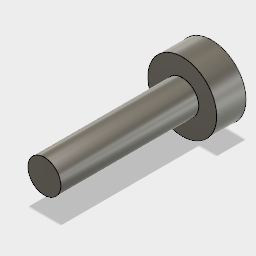
Spool_Holder_and_Filament_Guide (Autodesk Fusion 360 archive; units mm, degrees)
design "3mm with Washer - Loose Fit"
Autodesk Fusion 360 part; units mm, degrees
cylinder "CylinderPrimitive1" add diameter 7.5 height 3.2 placed x (1, 0, 0) y (0, 1, 0) z (0, 0, 1) at (0, 0, 0)
cylinder "CylinderPrimitive2" add diameter 3.6 height 15 placed x (1, 0, 0) y (0, 1, 0) z (0, 0, 1) at (0, 0, 3.2)

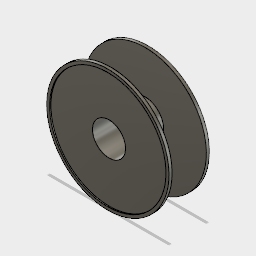
design "Spool"
Autodesk Fusion 360 part; units mm, degrees
sketch "Spool" plane through (0, 0, 0) normal (1, 0, 0) x (0, 0, -1)
  line L0 (33, -100) -> (28, -100)
  line L1 (28, -100) -> (28, -30)
  line L2 (10, 0) -> (0, 0) construction
  line L3 (33, -100) -> (33, -95)
  line L4 (33, -95) -> (31, -95)
  line L5 (31, -95) -> (31, -27)
  line L6 (0, -27) -> (0, -87.6876) construction
  line L7 (0, -27) -> (31, -27)
  line L8 (28, -30) -> (0, -30)
  line L9 (-33, -100) -> (-28, -100)
  line L10 (-28, -100) -> (-28, -30)
  line L11 (-28, -30) -> (0, -30)
  line L12 (0, -27) -> (-31, -27)
  line L13 (-31, -95) -> (-31, -27)
  line L14 (-33, -100) -> (-33, -95)
  line L15 (-33, -95) -> (-31, -95)
  line L16 (0, 10) -> (0, 0) construction
  dimension "d17" = 5
  dimension "d18" = 100
  dimension "d20" = 27
  dimension "d24" = 28
  dimension "d37" = 3
  dimension "d44" = 33
  dimension "d46" = 2
  measures "d17" distance of L0.start L3.end
  measures "d18" distance of L0 L2
  measures "d20" distance of L2 L7
  measures "d24" distance of L1 L6
  measures "d37" distance of L7 L8
  measures "d44" distance of L3 L6
  measures "d46" distance of L3 L5
revolve "Revolve1" add sketch "Spool" angle 360 about axis through (0, 0, -10) along (0, 0, 1)
ref_plane "WorkPlane1" through (0, 0, 0) normal (0, 0, 1) x (1, 0, 0)
equation "d18 = 0.5 * SpoolDia"
equation "d20 = 0.5 * HubDia"
equation "d24 = 0.5 * InsideHeight"
equation "d37 = Thickness"
equation "SpoolDia = 200 mm"
equation "HubDia = 54 mm"
equation "TotalHeight = 66 mm"
equation "d44 = 0.5 * TotalHeight"
equation "LipSize = 2 mm"
equation "d46 = LipSize"
equation "InsideHeight = 56 mm"
equation "Thickness = 0.5 * ( TotalHeight - InsideHeight ) - LipSize"
named bodies: "Spool"

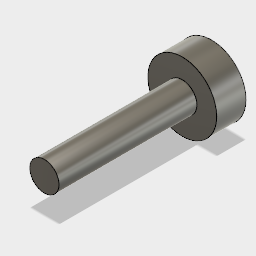
design "3mm with Washer - Close Fit"
Autodesk Fusion 360 part; units mm, degrees
cylinder "CylinderPrimitive1" add diameter 7.5 height 3.2 placed x (1, 0, 0) y (0, 1, 0) z (0, 0, 1) at (0, 0, 0)
cylinder "CylinderPrimitive2" add diameter 3.2 height 15 placed x (1, 0, 0) y (0, 1, 0) z (0, 0, 1) at (0, 0, 3.2)

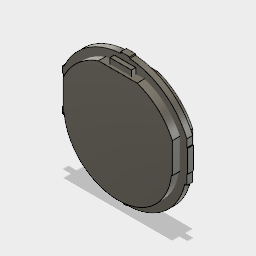
design "RFID Reader Cut Out"
Autodesk Fusion 360 part; units mm, degrees
ref_plane "WorkPlane1" through (3.9732, 4.9722, 0) normal (0, 0, 1) x (1, 0, 0)
sketch "Body Cut for Electronics" plane through (0, 0, 0) normal (0, 0, 1) x (1, 0, 0)
  line L0 (2.1432, 29.163) -> (5.5032, 29.163)
  line L1 (3.8232, 29.163) -> (3.8232, 19.163) construction
  line L2 (7.8232, 29.163) -> (7.8232, 19.163)
  line L3 (-0.1768, 19.163) -> (7.8232, 19.163)
  line L4 (2.1432, 29.163) -> (2.1432, 28.6377)
  line L5 (5.5032, 29.163) -> (5.5032, 28.6548)
  arc A0 (26.7732, 13.4919) -> (5.5032, 28.6548) centre (3.8232, 3.7982) ccw
  arc A1 (2.1432, 28.6377) -> (-18.9127, 13.9615) centre (3.8256, 3.7813) ccw
  line L6 (-0.1768, 26.913) -> (7.8232, 26.913)
  line L7 (-0.1768, 29.163) -> (-0.1768, 19.163)
  dimension "d10" = 10
  dimension "d11" = 4
  measures "d10" distance of L1.start L1.end
sketch "sketch 149" plane through (0, 0, 0) normal (0, 0, 1) x (1, 0, 0)
  line L0 (2.1432, 29.163) -> (2.1432, 28.6377)
  line L1 (5.5032, 29.163) -> (5.5032, 28.6548)
  line L2 (26.7732, 13.4919) -> (26.7732, 10.6115)
  line L3 (26.7732, 2.2615) -> (26.7732, -1.4856)
  line L4 (27.0732, 10.6115) -> (27.0732, 2.2615)
  line L5 (3.0732, -19.1885) -> (3.0732, -18.9361)
  line L6 (4.5732, -19.1885) -> (4.5732, -18.9374)
  line L7 (27.0732, 10.6115) -> (26.7732, 10.6115)
  arc A0 (26.7732, 13.4919) -> (5.5032, 28.6548) centre (3.8232, 3.7982) ccw
  arc A1 (2.1432, 28.6377) -> (-18.9127, 13.9615) centre (3.8256, 3.7813) ccw
  line L8 (27.0732, 2.2615) -> (26.7732, 2.2615)
  arc A2 (-18.2279, -1.5385) -> (3.0732, -18.9361) centre (3.4131, 3.2191) ccw
  arc A3 (4.5732, -18.9374) -> (25.986, -1.4856) centre (4.3334, 3.2191) ccw
  line L9 (2.1432, 29.163) -> (5.5032, 29.163)
  line L10 (3.0732, -19.1885) -> (4.5732, -19.1885)
  arc A4 (26.6232, 13.4615) -> (5.2532, 28.5202) centre (3.8232, 3.7982) ccw construction
  line L11 (26.7732, -1.4856) -> (25.986, -1.4856)
  line L12 (-19.4268, -1.5385) -> (-18.2279, -1.5385)
  line L13 (-19.4268, 1) -> (-19.1268, 1)
  line L14 (-19.1268, 11.4615) -> (-19.1268, 1)
  line L15 (-19.4268, 1) -> (-19.4268, -1.5385)
  line L16 (4.3232, -19.0385) -> (4.3232, -18.7872) construction
  line L17 (3.3232, -19.0385) -> (4.3232, -19.0385) construction
  line L18 (-18.9768, 13.4615) -> (-18.9768, -0.7885) construction
  line L19 (-18.9768, 13.4615) -> (-18.9768, -0.7885) construction
  line L20 (-18.9768, -0.7885) -> (-18.3268, -0.7885) construction
  line L21 (-19.4268, 13.9615) -> (-18.9127, 13.9615)
  line L22 (-19.4268, 11.4615) -> (-19.1268, 11.4615)
  line L23 (-19.4268, 13.9615) -> (-19.4268, 11.4615)
  line L24 (5.2532, 28.983) -> (5.2532, 28.5202) construction
  line L25 (2.3932, 28.983) -> (2.3932, 28.5202) construction
  line L26 (2.3932, 28.983) -> (5.2532, 28.983) construction
  line L27 (3.8232, 28.983) -> (3.8232, -21) construction
extrude "Extrude1" add sketch "sketch 149" along normal blind 1 and the other way blind 1 makes body 1
extrude "Extrude3" add sketch "Body Cut for Electronics" along normal blind 2.5 contours L2 L3 L6 L7 bodies 1
sketch "sketch 214" plane through (0, 0, 0) normal (0, 0, 1) x (1, 0, 0)
  line L0 (24.1232, 12.9395) -> (24.1232, 1.7115)
  line L1 (24.1232, 1.7115) -> (23.7829, 1.7115)
  line L2 (-16.4768, 1.7115) -> (-16.1364, 1.7115)
  line L3 (-16.4768, 12.9395) -> (-16.4768, 1.7115)
  arc A0 (24.1232, 12.9395) -> (-16.4768, 12.9395) centre (3.8232, 3.7982) ccw
  arc A1 (-16.1364, 1.7115) -> (23.7829, 1.7115) centre (3.8232, 3.785) ccw
  line L4 (-9.1914, 24.8657) -> (16.8378, 24.8657)
extrude "Extrude2" add sketch "sketch 214" along normal blind 3.5 and the other way blind 3.5 separate body contours L0 L1 L2 L3 A0 A1 L4 makes body 2
scale "Scale1" factors (1.0105, 1.014, 1.1) about (3.8232, 4.8657, 0) bodies 1 2
named bodies: "RFID Cavity", "Through Cut"
